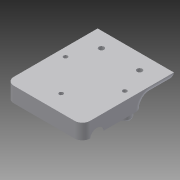
# Autodesk Inventor part: 137 V Dipole Bottom
Saved by Autodesk Inventor 2014 (Build 180170000, 170)
## iProperties
Created: 2023-07-11
Part Number: 137 V Dipole Bottom
Material: Generic
Document SubType Name: Modeling
Designer: VMUser
Density: 1 g/cm^3
Appearance: Default
Author: VMUser
Autodesk Inventor part; units mm, degrees
ref_plane "YZ Plane" through (0, 0, 0) normal (1, 0, 0) x (0, 1, 0)
sketch "Sketch1" plane through (0, 0, 0) normal (0, 1, 0) x (-1, 0, 0)
  line L0 (0, 0) -> (63.5, 0)
  line L1 (63.5, 0) -> (63.5, -50.8)
  line L2 (63.5, -50.8) -> (0, -50.8)
  line L3 (0, -50.8) -> (0, 0)
  line L4 (31.75, -50.8) -> (31.75, -30.48)
  line L5 (31.75, -30.48) -> (63.5, -12.1491)
  line L6 (31.75, -30.48) -> (0, -12.1491)
  line L7 (31.75, -30.48) -> (68.4117, -30.48) construction
  dimension "d0" = 63.5
  dimension "d1" = 50.8
  dimension "d2" = 20.32
  dimension "d3" = 120
  dimension "d4" = 150
  dimension "d5" = 120
  constraints: 16 end point, 3 parallel, 2 horizontal, 2 point on line, 1 equal length, 1 midpoint, 1 perpendicular
  measures "d0" distance of L1.end L2.end
  measures "d1" distance of L0.end L1.end
  measures "d2" distance of L4.start L4.end
  measures "d3" angle of L4 L5
  measures "d4" angle of L7 L6
  measures "d5" angle of L5 L6
extrude "Extrusion1" add sketch "Sketch1" along normal blind 12.7
ref_plane "Work Plane1" through (0, 0, 0) normal (0.8660254, 0, 0.5) x (0, 1, 0)
ref_plane "Work Plane2" through (-31.75, 0, -50.8) normal (-1, 0, 0) x (0, 0, 1)
sketch "Sketch2" plane through (0, 0, 0) normal (0.8660254, 0, 0.5) x (0, 1, 0)
  circle A0 centre (0, -10.5215) radius 4.826
  point P0 (0, 0)
  point P1 (0, -10.5215)
  dimension "d10" = 9.652
  constraints: 1 centre point, 1 coincident
  measures "d10" diameter of A0
extrude "Extrusion2" cut sketch "Sketch2" against normal up to surface surface through (-31.75, 0, -50.8) normal (-1, 0, 0)
mirror "Mirror2" about plane through (-31.75, 0, -50.8) normal (-1, 0, 0) of "Extrusion2"
sketch "Sketch5" plane through (0, 0, -50.8) normal (0, 0, -1) x (-1, 0, 0)
  circle A0 centre (31.75, 0) radius 3.556
  dimension "d18" = 7.112
  constraints: 1 centre point, 1 coincident
  measures "d18" diameter of A0
extrude "Extrusion4" cut sketch "Sketch5" against normal blind 20.32
sketch "Sketch6" plane through (0, 0, 0) normal (0, -1, 0) x (1, 0, 0)
  line L0 (-35.306, -33.9995) -> (-63.5, -17.7217) projected
  circle A0 centre (-60.2004, -19.6267) radius 1.3335
  line L1 (14.7857, -57.3474) -> (-82.6851, -1.0726) projected
  point P0 (0, 0)
  dimension "d21" = 2.667
  dimension "d23" = 1.905
  constraints: 1 centre point, 1 point on line
  measures "d21" diameter of A0
  measures "d23" vertical distance of L0.end A0.centre
revolve "Revolution1" cut sketch "Sketch6" angle 360 about axis through (-68.7607, 0, -9.1118) along (-0.8660254, 0, 0.5)
mirror "Mirror3" about plane through (-31.75, 0, -50.8) normal (-1, 0, 0) of "Revolution1"
sketch "Sketch11" plane through (0, 0, 0) normal (0, -1, 0) x (1, 0, 0)
  line L0 (-35.306, -50.8) -> (-35.306, -33.9995) projected
  circle A0 centre (-35.306, -42.3998) radius 1.016
  line L1 (-31.75, -60.96) -> (-31.75, 10.16) projected
  point P0 (0, 0)
  dimension "d33" = 2.032
  constraints: 1 centre point, 1 midpoint
  measures "d33" diameter of A0
revolve "Revolution4" cut sketch "Sketch11" angle 360 about axis through (-31.75, 0, -50.8) along (0, 0, 1)
sketch "Sketch12" plane through (0, 0, 0) normal (0, -1, 0) x (1, 0, 0)
  arc A0 (-6.9707, -10.6011) -> (-9.2804, -11.9346) centre (-8.1256, -11.2678) ccw projected
  arc A1 (-54.2196, -11.9346) -> (-56.5293, -10.6011) centre (-55.3744, -11.2678) ccw projected
  arc A2 (-9.3141, -10.6632) -> (-54.1859, -10.6632) centre (-31.75, -56.2403) ccw
  arc A3 (-9.4587, -11.3001) -> (-54.0413, -11.3001) centre (-31.75, -56.2403) ccw
  arc A4 (-8.881, -10.169) -> (-54.619, -10.169) centre (-31.75, -56.2403) ccw
  dimension "d35" = 50.8
  dimension "d36" = 0.635
  dimension "d37" = 0.635
  constraints: 12 point on circle, 3 centre point
  measures "d35" radius of A2
  measures "d36" radial gap between concentric circles of A4 A2
  measures "d37" radial gap between concentric circles of A2 A3
extrude "Extrusion5" cut sketch "Sketch12" against normal blind 1.27
sketch "Sketch13" plane through (0, 0, 0) normal (0, -1, 0) x (1, 0, 0)
  arc A0 (-35.306, -41.3838) -> (-35.306, -43.4158) centre (-35.306, -42.3998) ccw projected
  arc A1 (-61.3553, -18.96) -> (-59.0456, -20.2935) centre (-60.2004, -19.6267) ccw projected
  arc A2 (-59.8182, -20.9043) -> (-36.3024, -42.2011) centre (-29.5982, -11.167) ccw
  arc A3 (-60.4761, -20.9314) -> (-36.2063, -42.8707) centre (-29.5982, -11.167) ccw
  arc A4 (-59.2583, -20.5704) -> (-35.9624, -41.6242) centre (-29.5982, -11.167) ccw
  point P0 (0, 0)
  dimension "d40" = 31.75
  dimension "d41" = 0.635
  dimension "d42" = 0.635
  constraints: 12 point on circle, 3 centre point
  measures "d40" radius of A2
  measures "d41" radial gap between concentric circles of A4 A2
  measures "d42" radial gap between concentric circles of A2 A3
extrude "Extrusion6" cut sketch "Sketch13" against normal blind 1.27
mirror "Mirror4" about plane through (-31.75, 0, -50.8) normal (-1, 0, 0) of "Extrusion6"
sketch "Sketch14" plane through (0, 0, 0) normal (0, -1, 0) x (1, 0, 0)
  arc A0 (-9.4587, -11.3001) -> (-54.0413, -11.3001) centre (-31.75, -56.2403) ccw projected
  arc A1 (-54.2196, -11.9346) -> (-54.0413, -11.3001) centre (-55.3744, -11.2678) ccw projected
  line L0 (-54.2196, -11.9346) -> (-31.75, -24.9074) projected
  line L1 (-31.75, -24.9074) -> (-9.2804, -11.9346) projected
  arc A2 (-9.4587, -11.3001) -> (-9.2804, -11.9346) centre (-8.1256, -11.2678) ccw projected
  arc A3 (-35.9624, -41.6242) -> (-36.2063, -42.8707) centre (-35.306, -42.3998) ccw projected
  arc A4 (-27.2937, -42.8707) -> (-27.5376, -41.6242) centre (-28.194, -42.3998) ccw projected
  line L2 (-35.306, -42.3998) -> (-56.388, -42.3998) construction
  line L3 (-31.75, -34.2474) -> (-31.75, -30.48) construction
  point P0 (0, 0)
  point P1 (-31.75, -14.1124)
  point P2 (-7.112, -42.3998)
  dimension "d45" = 10.795
  dimension "d46" = 21.082
  constraints: 2 end point, 1 coincident, 1 horizontal, 1 symmetric about line
  measures "d45" distance of L0.end point (-31.75, -14.112)
  measures "d46" distance of L2.start L2.end
sketch "Sketch15" plane through (0, 0, 0) normal (0, -1, 0) x (1, 0, 0)
  circle A0 centre (-31.75, -14.1124) radius 5.08
  circle A1 centre (-56.388, -42.3998) radius 5.08
  circle A2 centre (-7.112, -42.3998) radius 5.08
  point P0 (0, 0)
  dimension "d47" = 10.16
  dimension "d48" = 10.16
  dimension "d49" = 10.16
  constraints: 3 centre point, 3 coincident
  measures "d47" diameter of A0
  measures "d48" diameter of A1
  measures "d49" diameter of A2
extrude "Extrusion7" add sketch "Sketch15" along normal blind 6.223
sketch "Sketch16" plane through (0, 12.7, 0) normal (0, 1, 0) x (1, 0, 0)
  circle A0 centre (-56.388, 42.3998) radius 5.08 projected
  circle A1 centre (-31.75, 14.1124) radius 5.08 projected
  circle A2 centre (-7.112, 42.3998) radius 5.08 projected
  circle A3 centre (-7.112, 42.3998) radius 5.08 projected
  constraints: 3 coincident
hole "Hole1" at (-56.388, 12.7, -42.3998) at (-31.75, 12.7, -14.1124) at (-7.112, 12.7, -42.3998) direction (0, -1, 0) diameter 3.4544 end through all
fillet "Fillet1" radius 1.5875 3 edges at (-36.83, -6.223, -14.1124) (-12.192, -6.223, -42.3998) (-61.468, -6.223, -42.3998)
sketch "Sketch17" plane through (0, 0, 0) normal (0, -1, 0) x (1, 0, 0)
  line L0 (-54.2196, -11.9346) -> (-31.75, -24.9074) projected
  line L1 (-31.75, -24.9074) -> (-33.9497, -23.6374)
  line L2 (-33.9497, -23.6374) -> (-34.7435, -25.0122)
  line L3 (-34.7435, -25.0122) -> (-32.5438, -26.2822)
  line L4 (-32.5438, -26.2822) -> (-31.75, -24.9074)
  line L5 (17.6126, -58.9795) -> (-83.1563, -0.8006) projected
  point P0 (0, 0)
  dimension "d60" = 2.54
  dimension "d61" = 1.5875
  constraints: 8 end point, 2 parallel, 1 perpendicular, 1 point on line
  measures "d60" distance of L0.end L1.end
  measures "d61" distance of L2.end L1.end
revolve "Revolution5" add sketch "Sketch17" angle 180 about axis through (-68.7607, 0, -9.1118) along (-0.8660254, 0, 0.5)
mirror "Mirror5" about plane through (-31.75, 0, -50.8) normal (-1, 0, 0) of "Revolution5"
sketch "Sketch18" plane through (0, 12.7, -50.8) normal (0, 0, -1) x (-1, 0, 0)
  line L0 (0, -12.7) -> (0, 0) projected
  line L1 (63.5, 0) -> (0, 0)
  line L2 (0, 0) -> (0, -6.35)
  line L3 (0, -6.35) -> (63.5, -6.35)
  line L4 (63.5, -6.35) -> (63.5, 0)
  constraints: 8 end point, 2 parallel, 1 horizontal, 1 midpoint, 1 perpendicular
extrude "Extrusion8" add sketch "Sketch18" along normal blind 25.4
fillet "Fillet2" radius 6.35 1 edges at (-31.75, 6.35, -50.8)
fillet "Fillet3" radius 6.35 5 edges at (-63.5, 4.4901, -52.6599) (-63.5, 6.35, -66.675) (-31.75, 6.35, -76.2) (0, 4.4901, -52.6599) (0, 6.35, -66.675)
fillet "Fillet4" radius 6.35 2 edges at (0, 6.35, 0) (-63.5, 6.35, 0)
sketch "Sketch19" plane through (-57.15, 6.35, -57.15) normal (0, -1, 0) x (1, 0, 0)
  line L0 (50.8, 0) -> (50.8, -12.7) projected
  line L1 (0, -12.7) -> (0, 0) projected
  point P0 (57.15, 57.15)
  point P1 (9.525, -6.35)
  point P2 (41.275, -6.35)
  dimension "d68" = 9.525
  dimension "d69" = 9.525
  measures "d68" distance from line of L1 point (9.525, -6.35)
  measures "d69" distance from line of L0 point (41.275, -6.35)
hole "Hole2" at (-47.625, 6.35, -63.5) at (-15.875, 6.35, -63.5) direction (0, 1, 0) diameter 4.3942 end through all
body "Solid1"
